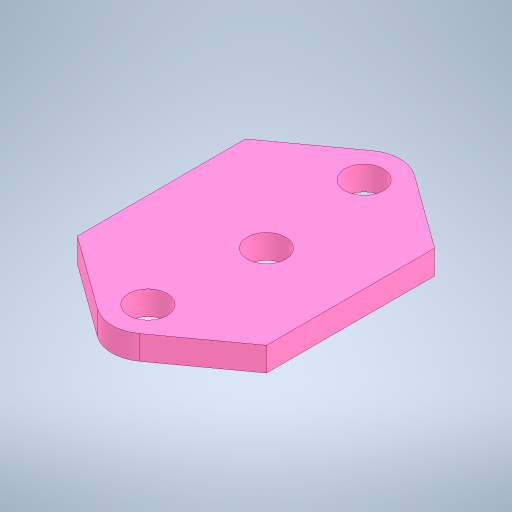
# Autodesk Inventor part: креп_отп_каретка
Saved by Autodesk Inventor 2023.1 (Build 271208000, 208)
## iProperties
Created: 2026-02-03
Part Number: креп_отп_каретка
Material: Типовые
Document SubType Name: Modeling
Designer: DELL
Density: 1 g/cm^3
Appearance: Розовый
Author: DELL
Autodesk Inventor part; units mm, degrees
ref_plane "YZ Plane" through (0, 0, 0) normal (1, 0, 0) x (0, 1, 0)
ref_plane "XZ Plane" through (0, 0, 0) normal (0, 1, 0) x (-1, 0, 0)
ref_plane "XY Plane" through (0, 0, 0) normal (0, 0, 1) x (1, 0, 0)
sketch "Эскиз1" plane through (0, 0, 0) normal (0, 1, 0) x (-1, 0, 0)
  line L0 (-15.75, 7) -> (15.75, 7) construction
  line L1 (15.75, 7) -> (15.75, -7) construction
  line L2 (15.75, -7) -> (-15.75, -7) construction
  line L3 (-15.75, -7) -> (-15.75, 7) construction
  line L4 (-15.75, 7) -> (15.75, -7) construction
  line L5 (15.75, 7) -> (-15.75, -7) construction
  line L6 (0, 7) -> (-15.75, 7)
  line L7 (-15.75, 7) -> (-15.75, -7)
  line L8 (-15.75, -7) -> (0, -7)
  line L9 (0, -7) -> (0, 7)
  circle A0 centre (-8.75, 0) radius 1.6
  point P0 (0, 0)
  dimension "d0" = 31.5
  dimension "d1" = 14
  dimension "d2" = 3.2
  dimension "d3" = 7
  constraints: 20 end point, 4 parallel, 3 midpoint, 2 horizontal, 2 perpendicular, 1 centre point
  measures "d0" distance of L1.end L2.end
  measures "d1" distance of L0.end L1.end
  measures "d2" diameter of A0
  measures "d3" distance from line of L3 A0.centre
extrude "Выдавливание1" add sketch "Эскиз1" along normal blind 2
sketch "Эскиз2" plane through (0, 2, 0) normal (0, 1, 0) x (1, 0, 0)
  circle A0 centre (8.75, 0) radius 1.6 projected
  circle A1 centre (7.875, 9) radius 1.6
  circle A2 centre (7.875, -9) radius 1.6
  line L0 (0, -7) -> (15.75, -7) projected
  line L1 (15.75, 7) -> (0, 7) projected
  circle A3 centre (7.875, -9) radius 3
  circle A4 centre (7.875, 9) radius 3
  line L2 (0, 7) -> (6.1151, 11.4296)
  line L3 (9.6349, 11.4296) -> (15.75, 7)
  line L4 (15.75, -7) -> (15.75, 7) projected
  line L5 (0, 7) -> (0, -7) projected
  line L6 (0, -7) -> (6.1151, -11.4296)
  line L7 (15.75, -7) -> (9.6349, -11.4296)
  line L8 (7.875, 9) -> (7.875, -16.4074) construction
  point P0 (0, 0)
  point P1 (5.8526, -11.2158)
  point P2 (8.7863, -11.8582)
  point P3 (10.1111, -7)
  point P4 (5.6389, -7)
  dimension "d6" = 3.2
  dimension "d7" = 3.2
  dimension "d9" = 2
  dimension "d10" = 6
  dimension "d11" = 6
  dimension "d14" = 2
  constraints: 10 end point, 6 point on circle, 4 centre point, 4 tangent, 2 coincident, 1 equal length, 1 point on line, 1 vertical
  measures "d6" diameter of A1
  measures "d7" diameter of A2
  measures "d9" distance from line of L1 A1.centre
  measures "d10" diameter of A3
  measures "d11" diameter of A4
  measures "d14" distance from line of L0 A2.centre
extrude "Выдавливание2" add sketch "Эскиз2" against normal blind 2 contours L0 A3 L6 | A3 L0 | L0 A3 | L2 A4 L1 | L0 L7 A3 | A4 L1 | A4 L3 L1 picked at (7.8107, 7.1372)
